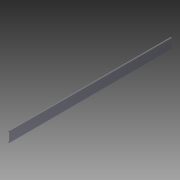
# Autodesk Inventor part: slide outer
Saved by Autodesk Inventor 2012 (Build 160160000, 160)
## iProperties
Created: 2011-12-02
Part Number: slide outer
Material: Steel
Document SubType Name: Modeling
Designer: Antonella
Mass: 100.774 g
Surface Area: 331.285 cm^2
Volume: 12.8375 cm^3
Density: 7.85 g/cm^3
Author: Antonella
Autodesk Inventor part; units mm, degrees
ref_plane "YZ Plane" through (0, 0, 0) normal (1, 0, 0) x (0, 1, 0)
ref_plane "XZ Plane" through (0, 0, 0) normal (0, 1, 0) x (-1, 0, 0)
ref_plane "XY Plane" through (0, 0, 0) normal (0, 0, 1) x (1, 0, 0)
sketch "Sketch1" plane through (0, 0, 0) normal (0, 0, 1) x (1, 0, 0)
  line L0 (-0.7938, 0) -> (4.7625, 0) projected
  line L1 (0, -20.5581) -> (0, 20.5581) projected
  line L2 (3.9688, 12.7) -> (3.9688, -12.7)
  arc A0 (3.9688, 12.7) -> (0, 12.7) centre (1.9844, 12.7) ccw
  arc A1 (0, -12.7) -> (3.9688, -12.7) centre (1.9844, -12.7) ccw
  arc A2 (0.7938, -12.7) -> (3.175, -12.7) centre (1.9844, -12.7) ccw
  line L3 (3.175, -12.7) -> (3.175, 12.7)
  arc A3 (3.175, 12.7) -> (0.7938, 12.7) centre (1.9844, 12.7) ccw
  line L4 (0, 12.7) -> (0.7938, 12.7)
  line L5 (0.7938, -12.7) -> (0, -12.7)
  line L6 (0, -12.7) -> (0, 12.7) construction
  point P0 (0, 0)
  point P1 (3.9688, 0)
  dimension "d0" = 0.7937
  dimension "d1" = 3.9688
  dimension "d2" = 25.4
  constraints: 10 end point, 8 point on circle, 6 tangent, 4 centre point, 2 parallel, 2 point on line, 1 collinear, 1 horizontal alignment, 1 midpoint, 1 perpendicular, 2 other
  measures "d0" distance between parallel lines of L2 L3
  measures "d1" distance between parallel lines of L1 L2
  measures "d2" distance between parallel lines of L4 L5
extrude "Extrusion1" add sketch "Sketch1" along normal mid plane 457.2 contours L3 A3 L4 A0 L2 L0 | L0 L2 A1 L5 A2 L3
body "Solid1"
